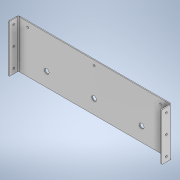
# Autodesk Inventor part: Platform side 2
Saved by Autodesk Inventor 2020 (Build 240168000, 168)
## iProperties
Created: 2022-07-05
Part Number: Platform side 2
Material: Generic
Document SubType Name: Sheet Metal
Designer: karimi2
Density: 1 g/cm^3
Sheet Metal Rule: Default_mm
Appearance: Aluminum - Dark
Author: karimi2
Autodesk Inventor part; units mm, degrees
ref_plane "YZ Plane" through (0, 0, 0) normal (1, 0, 0) x (0, 1, 0)
ref_plane "XZ Plane" through (0, 0, 0) normal (0, 1, 0) x (-1, 0, 0)
ref_plane "XY Plane" through (0, 0, 0) normal (0, 0, 1) x (1, 0, 0)
sketch "Sketch1" plane through (0, 0, 0) normal (0, 0, 1) x (1, 0, 0)
  line L0 (180, -50) -> (-180, -50)
  line L1 (-180, -50) -> (-180, 50)
  line L2 (-180, 50) -> (180, 50)
  line L3 (180, 50) -> (180, -50)
  circle A0 centre (-100, -20) radius 5
  circle A1 centre (0, -20) radius 5
  circle A2 centre (100, -20) radius 5
  circle A3 centre (-170, 40) radius 2
  circle A4 centre (-170, 0) radius 2
  circle A5 centre (-170, -40) radius 2
  circle A6 centre (170, 40) radius 2
  circle A7 centre (170, 0) radius 2
  circle A8 centre (170, -40) radius 2
  circle A9 centre (-140, 40) radius 2
  circle A10 centre (0, 40) radius 2
  circle A11 centre (140, 40) radius 2
  point P0 (0, 0)
  point P1 (0, 0)
  dimension "d4" = 10
  dimension "d13" = 360
  dimension "d14" = 180
  dimension "d15" = 100
  dimension "d16" = 10
  dimension "d17" = 10
  dimension "d18" = 30
  dimension "d19" = 80
  dimension "d20" = 10
  dimension "d21" = 10
  dimension "d22" = 4
  dimension "d23" = 50
  dimension "d24" = 10
  dimension "d25" = 50
  dimension "d26" = 80
  dimension "d27" = 70
  dimension "d28" = 180
  dimension "d29" = 180
  dimension "d47" = 40
  dimension "d48" = 40
  dimension "d49" = 4
  constraints: 12 centre point, 9 equal radius, 8 end point, 8 horizontal alignment, 4 vertical alignment, 2 parallel, 1 horizontal, 1 perpendicular
  measures "d4" diameter of A0
  measures "d13" distance of L1.end L2.end
  measures "d14" distance from line of point (0, 0) L1
  measures "d15" distance between parallel lines of L0 L2
  measures "d16" distance from line of L2 A3.centre
  measures "d17" distance from line of L1 A3.centre
  measures "d18" distance from line of L0 A0.centre
  measures "d19" distance from line of L1 A0.centre
  measures "d20" distance from line of L0 A5.centre
  measures "d21" distance from line of L1 A5.centre
  measures "d22" diameter of A6
  measures "d23" distance from line of point (0, 0) L2
  measures "d24" distance from line of A6.centre L3
  measures "d25" distance from line of A7.centre L2
  measures "d26" distance from line of A2.centre L3
  measures "d27" distance from line of A2.centre L2
  measures "d28" distance from line of point (0, 0) L3
  measures "d29" distance from line of A1.centre L3
  measures "d47" distance from line of L3 A11.centre
  measures "d48" distance from line of L1 A9.centre
  measures "d49" diameter of A9
extrude "Plate2" add sketch "Sketch1" along normal blind 2
sketch "Sketch4" plane through (0, 0, 2) normal (0, 0, 1) x (1, 0, 0)
  line L0 (-180, 50) -> (180, 50) projected
  line L1 (-160, 50) -> (-160, -50)
  line L2 (-180, -50) -> (-180, 50) projected
  point P0 (0, 0)
  dimension "d50" = 100
  dimension "d51" = 20
  constraints: 2 end point, 1 perpendicular, 1 point on line
  measures "d50" distance of L1.start L1.end
  measures "d51" distance between parallel lines of L2 L1
fold "Fold3" angle 90 bend radius 2 thickness 2 k factor 0.44 line from (-160, 50, 2) to (-160, -50, 2) line at bend centre moving side (-1, 0, 0) folds toward (0, 0, 1)
sketch "Sketch5" plane through (0, 0, 2) normal (0, 0, 1) x (1, 0, 0)
  line L0 (160, 50) -> (160, -50)
  line L1 (180, -50) -> (-157.7381, -50) projected
  line L2 (180, 50) -> (180, -50) projected
  point P0 (0, 0)
  dimension "d58" = 100
  dimension "d59" = 20
  constraints: 2 end point, 1 point on line, 1 vertical
  measures "d58" distance of L0.start L0.end
  measures "d59" distance between parallel lines of L2 L0
fold "Fold4" angle 90 bend radius 2 thickness 2 k factor 0.44 line from (160, 50, 2) to (160, -50, 2) line at bend centre moving side (1, 0, 0) folds toward (0, 0, 1)
fillet "Fillet1" radius 2 4 edges at (160.7381, 50, 21.7381) (160.7381, -50, 21.7381) (-160.7381, 50, 21.7381) (-160.7381, -50, 21.7381)
equation "\"d30\" = Thickness"
equation "\"d52\" = BendReliefWidth"
equation "\"d53\" = BendReliefDepth"
equation "\"d54\" = MinimumRemnant"
equation "\"d55\" = TransitionRadius"
equation "\"d57\" = BendRadius"
equation "\"d60\" = BendReliefWidth"
equation "\"d61\" = BendReliefDepth"
equation "\"d62\" = MinimumRemnant"
equation "\"d63\" = TransitionRadius"
equation "\"d65\" = BendRadius"
equation "\"BendRadius\" = Thickness"
equation "\"BendReliefWidth\" = Thickness"
equation "\"BendReliefDepth\" = 0.5 * Thickness"
equation "\"CornerReliefSize\" = 4 * Thickness"
equation "\"MinimumRemnant\" = 2 * Thickness"
equation "\"TransitionRadius\" = BendRadius"
equation "\"JacobiRadiusSize\" = BendRadius"
equation "\"GapSize\" = Thickness"
equation "\"Thickness\" = 2"
body "Solid1"
